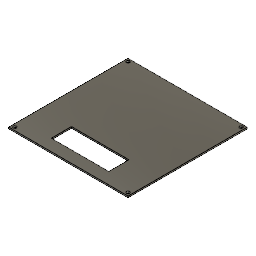
incubetter lid (Autodesk Fusion 360 design; units mm, degrees)
Autodesk Fusion 360 part; units mm, degrees
note: some values were not read from the file. Set by a fixed rule: which sketch regions a step uses.
sketch "Sketch1" plane through (0, 0, 0) normal (0, 0, 1) x (1, 0, 0)
  line L0 (75, 75) -> (-75, 75)
  line L1 (-75, 75) -> (-75, -75)
  line L2 (-75, -75) -> (75, -75)
  line L3 (75, -75) -> (75, 75)
  line L4 (75, 75) -> (-75, -75) construction
  line L5 (-75, 75) -> (75, -75) construction
  dimension "d1" = 150
  dimension "d2" = 150
extrude "Extrude1" add sketch "Sketch1" along normal blind 1
sketch "Sketch2" plane through (0, 0, 1) normal (0, 0, 1) x (-1, 0, 0)
  line L0 (-75, 75) -> (-75, -75)
  line L1 (-75, -75) -> (75, -75)
  line L2 (75, -75) -> (75, 75)
  line L3 (75, 75) -> (-75, 75)
  line L4 (-75, -75) -> (-71, -75)
  line L5 (-71, -75) -> (-71, -71)
  line L6 (-71, -71) -> (-75, -71)
  line L7 (-75, -71) -> (-75, -75)
  circle A0 centre (-71, -71) radius 2
  dimension "d5" = 4
  dimension "d6" = 4
  dimension "d7" = 4
  measures "d7" diameter of A0
extrude "Extrude2" cut sketch "Sketch2" against normal blind 1 contours L5 L6 A0 | L5 L6 A0
sketch "Sketch3" plane through (0, 0, 1) normal (0, 0, 1) x (-1, 0, 0)
  circle A0 centre (-71, -71) radius 2
  line L0 (-75, 75) -> (-75, -75)
  line L1 (-75, -75) -> (75, -75)
  line L2 (75, -75) -> (75, 75)
  line L3 (75, 75) -> (-75, 75)
  line L4 (75, -75) -> (71, -75)
  line L5 (71, -75) -> (71, -71)
  line L6 (71, -71) -> (75, -71)
  line L7 (75, -71) -> (75, -75)
  line L8 (75, 75) -> (71, 75)
  line L9 (71, 75) -> (71, 71)
  line L10 (71, 71) -> (75, 71)
  line L11 (75, 71) -> (75, 75)
  line L12 (-75, 75) -> (-71, 75)
  line L13 (-71, 75) -> (-71, 71)
  line L14 (-71, 71) -> (-75, 71)
  line L15 (-75, 71) -> (-75, 75)
  circle A1 centre (-71, 71) radius 2
  circle A2 centre (71, 71) radius 2
  circle A3 centre (71, -71) radius 2
  dimension "d10" = 4
  dimension "d11" = 4
  dimension "d12" = 4
  dimension "d13" = 4
  dimension "d14" = 4
  dimension "d15" = 4
  dimension "d16" = 4
  dimension "d17" = 4
  dimension "d18" = 4
  measures "d16" diameter of A1
  measures "d17" diameter of A2
  measures "d18" diameter of A3
extrude "Extrude3" cut sketch "Sketch3" against normal blind 1 contours L13 L14 A1 | L13 L14 A1 | L9 L10 A2 | L9 L10 A2 | L5 L6 A3 | L5 L6 A3
sketch "Sketch4" plane through (0, 0, 1) normal (0, 0, 1) x (-1, 0, 0)
  circle A0 centre (71, -71) radius 2
  circle A1 centre (71, 71) radius 2
  circle A2 centre (-71, 71) radius 2
  circle A3 centre (-71, -71) radius 2
  line L0 (-75, 75) -> (-75, -75)
  line L1 (-75, -75) -> (75, -75)
  line L2 (75, -75) -> (75, 75)
  line L3 (75, 75) -> (-75, 75)
  line L4 (0, 75) -> (0, 60)
  line L5 (0, 60) -> (-36, 60)
  line L6 (-36, 60) -> (36, 60)
  line L7 (36, 60) -> (36, 35)
  line L8 (36, 35) -> (-36, 35)
  line L9 (-36, 35) -> (-36, 60)
  dimension "d21" = 15
  dimension "d24" = 72
extrude "Extrude4" cut sketch "Sketch4" against normal blind 1 contours L5 L6 L7 L8 L9
extrude "Extrude5" add 1 faces at (-12, 35.1244, 1) along direction (0, 0, 1) blind 1
